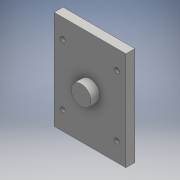
# Autodesk Inventor part: connectorModelFinal
Saved by Autodesk Inventor 2016 (Build 200138000, 138)
## iProperties
Created: 2017-02-16
Part Number: connectorModelFinal
Material: Generic
Document SubType Name: Modeling
Designer: 2boedeke
Density: 1 g/cm^3
Appearance: Default
Author: 2boedeke
Autodesk Inventor part; units mm, degrees
ref_plane "YZ Plane" through (0, 0, 0) normal (1, 0, 0) x (0, 1, 0)
ref_plane "XZ Plane" through (0, 0, 0) normal (0, 1, 0) x (-1, 0, 0)
ref_plane "XY Plane" through (0, 0, 0) normal (0, 0, 1) x (1, 0, 0)
sketch "Sketch1" plane through (0, 0, 0) normal (0, 1, 0) x (-1, 0, 0)
  line L0 (20, 27.5) -> (-20, 27.5)
  line L1 (-20, 27.5) -> (-20, -27.5)
  line L2 (-20, -27.5) -> (20, -27.5)
  line L3 (20, -27.5) -> (20, 27.5)
  circle A0 centre (15, 17) radius 1.35
  circle A1 centre (15, -17) radius 1.35
  circle A2 centre (-15, 17) radius 1.35
  circle A3 centre (-15, -17) radius 1.35
  point P0 (0, 0)
  dimension "d0" = 40
  dimension "d1" = 55
  dimension "d2" = 2.7
  dimension "d3" = 2.7
  dimension "d4" = 2.7
  dimension "d5" = 2.7
  constraints: 8 end point, 4 centre point, 2 parallel, 1 horizontal, 1 perpendicular
  measures "d0" distance of L2.end L1.end
  measures "d1" distance of L1.end L0.end
  measures "d2" diameter of A0
  measures "d3" diameter of A1
  measures "d4" diameter of A2
  measures "d5" diameter of A3
extrude "Extrusion1" add sketch "Sketch1" along normal blind 5
sketch "Sketch2" plane through (0, 0, 0) normal (0, -1, 0) x (1, 0, 0)
  circle A0 centre (0, 0) radius 5.5
  dimension "d8" = 11
  constraints: 1 centre point, 1 coincident
  measures "d8" diameter of A0
extrude "Extrusion2" add sketch "Sketch2" along normal blind 5
body "Solid1"
